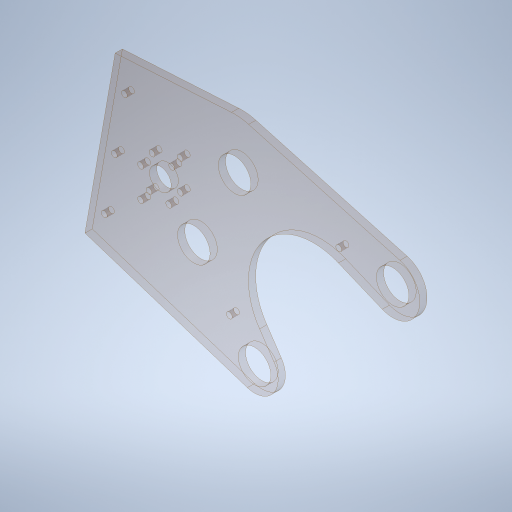
# Autodesk Inventor part: GP7-001
Saved by Autodesk Inventor 2023.4 (Build 274418000, 418)
## iProperties
Created: 2025-02-24
Part Number: GP7-001
Material: Polycarbonate, Smoke
Document SubType Name: Modeling
Designer: dlangdon
Density: 1.2 g/cm^3
Appearance: Polycarbonate - Smoked
Author: dlangdon
Autodesk Inventor part; units mm, degrees
ref_plane "YZ Plane" through (0, 0, 0) normal (1, 0, 0) x (0, 1, 0)
ref_plane "XZ Plane" through (0, 0, 0) normal (0, 1, 0) x (-1, 0, 0)
ref_plane "XY Plane" through (0, 0, 0) normal (0, 0, 1) x (1, 0, 0)
sketch "Sketch1" plane through (0, 0, 0) normal (0, 0, 1) x (1, 0, 0)
  circle A0 centre (65.1069, 65.1069) radius 38.1 construction
  circle A1 centre (-56.1266, -56.1266) radius 25.4 construction
  circle A2 centre (0, 0) radius 53.975 construction
  line L0 (-38.1661, -38.1661) -> (38.1661, 38.1661) construction
  line L1 (65.1069, 65.1069) -> (-56.1266, -56.1266) construction
  line L2 (-4.3707, 6.2419) -> (-4.3707, 53.7978) construction
  line L3 (-211.1644, -81.5266) -> (654.2277, -81.5266) construction
  circle A3 centre (163.556, -24.3766) radius 57.15 construction
  circle A4 centre (65.1069, 65.1069) radius 14.2875
  circle A5 centre (-56.1266, -56.1266) radius 14.2875
  circle A6 centre (-4.3707, 6.2419) radius 57.15 construction
  circle A7 centre (-56.1266, -56.1266) radius 20.6375 construction
  circle A8 centre (65.1069, 65.1069) radius 23.8125 construction
  circle A9 centre (-73.6972, 80.6773) radius 14.2875
  line L4 (-73.6972, 80.6773) -> (65.1069, 65.1069) construction
  circle A10 centre (65.1069, 65.1069) radius 14.3256 construction
  circle A11 centre (-56.1266, -56.1266) radius 14.3256 construction
  circle A12 centre (-109.5316, 9.8231) radius 14.2875
  line L5 (-56.1266, -56.1266) -> (-109.5316, 9.8231) construction
  circle A13 centre (-109.5316, 9.8231) radius 39.7002 construction
  circle A14 centre (-73.6972, 80.6773) radius 39.7002 construction
  line L6 (17.4877, 59.0466) -> (55.9992, 43.1049)
  line L7 (-39.0193, -44.5834) -> (-51.7448, -25.7239)
  arc A15 (17.4877, 59.0466) -> (-51.7448, -25.7239) centre (-4.3707, 6.2419) ccw
  line L8 (-178.6215, 120.6011) -> (-153.6074, 116.1905) construction
  line L9 (-153.6074, 116.1905) -> (-180.0714, -33.8943) construction
  line L10 (-180.0714, -33.8943) -> (-205.0855, -29.4836) construction
  line L11 (-205.0855, -29.4836) -> (-178.6215, 120.6011) construction
  line L12 (-209.5607, -54.8639) -> (55.1963, -101.5477) construction
  line L13 (-174.1463, 145.9814) -> (158.0246, 87.4107) construction
  line L14 (-174.1463, 145.9814) -> (-209.5607, -54.8639) construction
  circle A16 centre (-138.9335, 44.7481) radius 25.4 construction
  circle A17 centre (-138.9335, 44.7481) radius 5.9531 construction
  line L15 (-84.5475, -21.0298) -> (-72.1113, -36.3871) construction
  circle A18 centre (17.7787, 70.4159) radius 9.525 construction
  line L16 (-166.1144, 118.3958) -> (-192.5784, -31.6889) construction
  line L17 (-170.5251, 93.3817) -> (-188.1678, -6.6748) construction
  circle A19 centre (-138.9335, 44.7481) radius 17.4625 construction
  circle A20 centre (-138.9335, 44.7481) radius 9.525
  circle A21 centre (-73.6972, 80.6773) radius 46.0502 construction
  line L18 (-178.6215, 120.6011) -> (-76.4165, 126.6471)
  line L19 (-61.3431, 125.0394) -> (71.4951, 88.0465)
  line L20 (-62.4968, -75.7563) -> (-205.0855, -29.4836)
  line L21 (-178.6215, 120.6011) -> (-205.0855, -29.4836)
  arc A22 (-61.3431, 125.0394) -> (-76.4165, 126.6471) centre (-73.6972, 80.6773) ccw
  arc A23 (55.9992, 43.1049) -> (71.4951, 88.0465) centre (65.1069, 65.1069) ccw
  arc A24 (-62.4968, -75.7563) -> (-39.0193, -44.5834) centre (-56.1266, -56.1266) ccw
  line L22 (-138.9335, 44.7481) -> (-128.9174, 59.0525) construction
  line L23 (-121.633, 69.4558) -> (-156.234, 20.0404) construction
  circle A25 centre (-156.234, 20.0404) radius 4.7625 construction
  line L24 (0, 0) -> (-4.3707, 6.2419) construction
  point P0 (-191.8535, 45.5588)
  point P1 (-78.3294, -28.7084)
  point P2 (-179.3464, 43.3534)
  point P3 (-179.3464, 43.3534)
  point P4 (-146.3135, 60.5745)
  point P5 (-156.3295, 46.2701)
  point P6 (-148.9496, 30.4437)
  point P7 (-131.5535, 28.9217)
  point P8 (-121.5374, 43.2261)
  point P9 (-63.3695, 121.1474)
  dimension "d7" = 50.8
  dimension "d18" = 79.4004
  dimension "d34" = 34.925
  dimension "d3" = 45
  dimension "d4" = 0
  dimension "d8" = 107.95
  dimension "d9" = 28.575
  dimension "d10" = 76.2
  dimension "d11" = 114.3
  dimension "d12" = 114.3
  dimension "d13" = 6.35
  dimension "d14" = 9.525
  dimension "d15" = 139.6746
  dimension "d16" = 28.6512
  dimension "d17" = 84.8614
  dimension "d19" = 79.4004
  dimension "d22" = 25.4
  dimension "d23" = 152.4
  dimension "d26" = 203.9436
  dimension "d27" = 50.8
  dimension "d28" = 11.9062
  dimension "d29" = 51
  dimension "d30" = 171.45
  dimension "d31" = 10
  dimension "d32" = 19.05
  dimension "d33" = 101.6
  dimension "d35" = 19.05
  dimension "d36" = 6.35
  dimension "d37" = 34.925
  dimension "d40" = 360
  dimension "d43" = 25
  dimension "d44" = 9.525
  dimension "d55" = 80
  dimension "d56" = 7.62
  constraints: 50 end point, 23 centre point, 22 coincident, 19 point on circle, 13 tangent, 9 midpoint, 5 equal radius, 4 collinear, 4 parallel, 4 point on line, 2 horizontal, 1 concentric, 1 perpendicular, 1 vertical, 20 other
  measures "d3" angle of L2 L0
  measures "d4" distance between parallel lines of L0 L1
  measures "d8" diameter of A2
  measures "d9" diameter of A4
  measures "d10" diameter of A0
  measures "d11" diameter of A3
  measures "d12" diameter of A6
  measures "d13" radial gap between concentric circles of A5 A7
  measures "d14" radial gap between concentric circles of A4 A8
  measures "d15" distance of L4.start L4.end
  measures "d16" diameter of A10
  measures "d17" distance of L5.start L5.end
  measures "d19" diameter of A14
  measures "d22" distance of L9.end L10.end
  measures "d23" distance of L10.end L8.start
  measures "d26" distance of L13.start L12.start
  measures "d27" diameter of A16
  measures "d28" diameter of A17
  measures "d29" angle of L3 L5
  measures "d30" distance from line of point (0, 0) L9
  measures "d31" angle of L3 L12
  measures "d32" diameter of A18
  measures "d33" distance of L17.start L17.end
  measures "d35" diameter of A20
  measures "d36" radial gap between concentric circles of A14 A21
  measures "d37" vertical distance of L5.end A16.centre
  measures "d43" angle of L9 L22
  measures "d44" diameter of A25
  measures "d55" angle of L1 L24
  measures "d56" distance of L24.start L24.end
extrude "Extrusion1" add sketch "Sketch1" along normal blind 6.35
hole "Hole1" at (-78.3294, -28.7084, 0) at (17.7787, 70.4159, 0) at (-170.5251, 93.3817, 0) at (-179.3464, 43.3534, 0) at (-188.1678, -6.6748, 0) at (-128.9174, 59.0525, 0) at (-146.3135, 60.5745, 0) at (-156.3295, 46.2701, 0) at (-148.9496, 30.4437, 0) at (-131.5535, 28.9217, 0) at (-121.5374, 43.2261, 0) at (-121.633, 69.4558, 0) at (-156.234, 20.0404, 0) direction (0, 0, 1) diameter 5.1054 end through all clearance for "Flat Head Machine Screw (82)" size "#10" standard "Ansi Unified Screw Threads"
body "Solid1"
